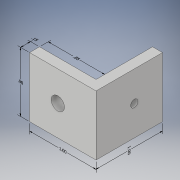
# Autodesk Inventor part: part v5
Saved by Autodesk Inventor 2018 (Build 220112000, 112)
## iProperties
Created: 2019-12-10
Part Number: part v5
Material: Generic
Document SubType Name: Modeling
Designer: AOFUser
Density: 1 g/cm^3
Appearance: Default
Author: AOFUser
Autodesk Inventor part; units mm, degrees
ref_plane "YZ Plane" through (0, 0, 0) normal (1, 0, 0) x (0, 1, 0)
ref_plane "XZ Plane" through (0, 0, 0) normal (0, 1, 0) x (-1, 0, 0)
ref_plane "XY Plane" through (0, 0, 0) normal (0, 0, 1) x (1, 0, 0)
sketch "Sketch1" plane through (0, 0, 0) normal (0, 1, 0) x (-1, 0, 0)
  line L0 (0, 0) -> (-25.4, 0)
  line L1 (-25.4, 0) -> (-25.4, -3.81)
  line L2 (-25.4, -3.81) -> (0, -3.81)
  line L3 (0, -3.81) -> (0, 0)
  line L4 (-25.4, 0) -> (-21.59, 0)
  line L5 (-21.59, 0) -> (-21.59, -25.4)
  line L6 (-21.59, -25.4) -> (-25.4, -25.4)
  line L7 (-25.4, -25.4) -> (-25.4, 0)
  dimension "d0" = 25.4
  dimension "d1" = 3.81
  dimension "d2" = 3.81
  dimension "d3" = 25.4
  constraints: 16 end point, 4 parallel, 2 horizontal, 2 perpendicular
  measures "d0" distance of L2.end L1.end
  measures "d1" distance of L1.end L0.end
  measures "d2" distance of L5.end L6.end
  measures "d3" distance of L4.end L5.end
extrude "Extrusion1" add sketch "Sketch1" along normal blind 22.86
sketch "Sketch2" plane through (21.59, 0, -25.4) normal (-1, 0, 0) x (0, 0, 1)
  line L0 (0, 0) -> (0, 22.86) projected
  line L1 (0, 11.43) -> (10.795, 11.43)
  point P0 (25.4, 0)
  dimension "d9" = 10.795
  constraints: 2 end point, 1 horizontal, 1 midpoint
  measures "d9" distance of L1.start L1.end
hole "Hole1" at (21.59, 11.43, -14.605) direction (1, 0, 0) diameter 2.794 end through all
sketch "Sketch3" plane through (21.59, 0, -3.81) normal (0, 0, -1) x (-1, 0, 0)
  line L0 (21.59, 0) -> (21.59, 22.86) projected
  line L1 (21.59, 11.43) -> (10.795, 11.43)
  dimension "d17" = 10.795
  constraints: 2 end point, 1 horizontal, 1 midpoint
  measures "d17" distance of L1.start L1.end
hole "Hole2" at (10.795, 11.43, -3.81) direction (0, 0, 1) diameter 5.08 end through all
body "Solid1"
